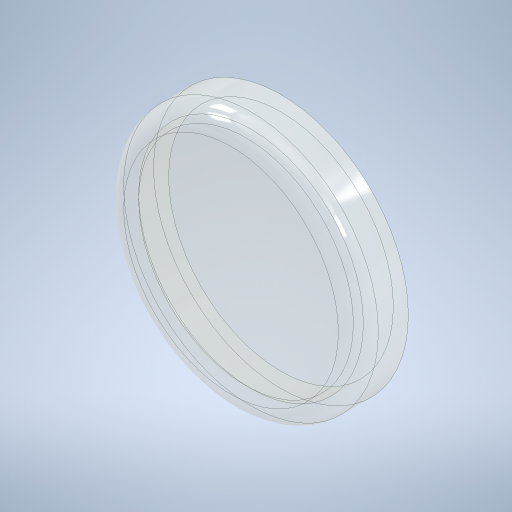
# Autodesk Inventor part: Buttonx26
Saved by Autodesk Inventor 2024 (Build 280153000, 153)
## iProperties
Created: 2023-09-15
Part Number: Buttonx26
Material: 玻璃
Document SubType Name: Modeling
Designer: nicx5
Density: 2.18 g/cm^3
Appearance: 透明
Author: nicx5
Autodesk Inventor part; units mm, degrees
ref_plane "YZ Plane" through (0, 0, 0) normal (1, 0, 0) x (0, 1, 0)
ref_plane "XZ Plane" through (0, 0, 0) normal (0, 1, 0) x (-1, 0, 0)
ref_plane "XY Plane" through (0, 0, 0) normal (0, 0, 1) x (1, 0, 0)
sketch "草图1" plane through (0, 0, 0) normal (0, 0, 1) x (1, 0, 0)
  circle A0 centre (0, 0) radius 12.75
  dimension "d0" = 25.5
  constraints: 1 centre point
  measures "d0" diameter of A0
extrude "拉伸1" add sketch "草图1" against normal blind 5
fillet "圆角1" radius 2 1 edges at (-12.75, 0, 0)
shell "抽壳1" thickness 1.5 removed faces 1 at (4.8553, -3.9738, -5)
